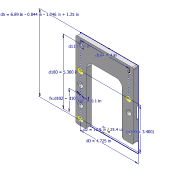
# Autodesk Inventor part: J002887
Saved by Autodesk Inventor 2012 SP2 (Build 160219200, 219)
## iProperties
Created: 2014-07-28
Material: ALUMINUM, 6061-T651
Vendor: HHMI: JFRC - ID&F
Document SubType Name: Modeling
Designer: arnoldj
Density: 2.7 g/cm^3
Part Number: J002887
Description: MPS Bottom Plate
Mass: 214.982 g
Surface Area: 270.982 cm^2
Volume: 79.623 cm^3
Project: P-194005
RuleStatus: InUse
AfterDocSave0: file://Part Number Cleaner
LAB/DEPT: SVOBODA (LAB)
REQUESTING SCIENTIST: PERON, SIMON
SURFACE ROUGHNESS: 63 Ra
DESIGN DEPARTMENT: HHMI: JFRC - ID&F
SPECIAL FINISH: ANODIZE PER MIL-A-8625F, TYPE II, CLASS 2 (BLACK)
ALTERED ITEM PART NUMBER: N/A
ALTERED ITEM VENDOR: N/A
ALTERED ITEM DESCRIPTION: N/A
Author: arnoldj
Revision Number: -
Autodesk Inventor part; units mm, degrees
ref_plane "Work Plane1 top of part" through (0, 0, 9.525) normal (0, 0, 1) x (1, 0, 0)
sketch "Sketch1" plane through (0, 0, 0) normal (0, 0, 1) x (1, 0, 0)
  line L0 (-60.0075, 146.25) -> (60.0075, 146.25)
  line L1 (60.0075, 146.25) -> (60.0075, -12.5)
  line L2 (-60.0075, -12.5) -> (-60.0075, 146.25)
  line L3 (-60.0075, -12.5) -> (60.0075, -12.5)
  point P0 (0, 0)
  point P1 (0, -3.5617)
  point P2 (0, 146.25)
  dimension "d0" = 120.015
  dimension "d2" = 12.5
  dimension "d5" = 158.75
  constraints: 8 end point, 2 perpendicular, 2 vertical alignment, 1 horizontal, 1 midpoint, 1 parallel
  measures "d0" distance of L1.end L2.start
  measures "d2" distance from line of L3 point (0, 0)
  measures "d5" distance of L2.start L0.start
extrude "Extrusion1" add sketch "Sketch1" along normal blind 9.525
sketch "Sketch2" plane through (0, 0, 0) normal (0, 0, 1) x (1, 0, 0)
  circle A0 centre (-50, 0) radius 3.175
  circle A1 centre (50, 86.36) radius 3.175
  circle A2 centre (-50, 86.36) radius 3.175
  point P0 (0, 0)
  point P1 (50, 35.56)
  dimension "d6" = 6.35
  dimension "d8" = 50
  dimension "d28" = 86.36
  dimension "d29" = 50
  dimension "d128" = 50.8
  constraints: 3 centre point, 1 equal radius, 1 horizontal alignment, 1 vertical alignment
  measures "d6" diameter of A0
  measures "d8" distance of point (0, 0) A0.centre
  measures "d28" distance of A0.centre A2.centre
  measures "d29" horizontal distance of point (0, 0) A1.centre
  measures "d128" distance of point (50, 35.56) A1.centre
hole "Hole1" at (-50, 0, 0) at (-50, 86.36, 0) at (50, 86.36, 0) direction (0, 0, 1) diameter 9.525 end through all
sketch "Sketch4" plane through (0, 0, 0) normal (0, 0, 1) x (1, 0, 0)
  line L0 (60.0075, -12.5) -> (-60.0075, -12.5) projected
  line L1 (0, 190.0524) -> (0, -46.2587) projected
  line L2 (-82.677, 0) -> (82.677, 0) projected
  line L3 (36.83, 110.944) -> (-36.83, 110.944)
  line L4 (-36.83, 110.944) -> (-36.83, -12.5)
  line L5 (36.83, 7.82) -> (60.0075, 7.82)
  line L6 (60.0075, 7.82) -> (60.0075, -12.5)
  line L7 (36.83, 7.82) -> (36.83, 110.944)
  line L8 (-36.83, -12.5) -> (60.0075, -12.5)
  line L9 (-60.0075, 146.25) -> (60.0075, 146.25) projected
  line L10 (0, -3.5649) -> (0, 156.2936)
  point P0 (0, 0)
  dimension "d30" = 123.444
  dimension "d31" = 20.32
  dimension "d32" = 35.306
  dimension "d112" = 73.66
  dimension "d132" = 36.83
  dimension "d133" = 36.83
  constraints: 14 end point, 3 point on line, 2 perpendicular, 1 collinear, 1 parallel, 1 symmetric about line
  measures "d30" distance of L3.end L4.end
  measures "d31" distance between parallel lines of L0 L5
  measures "d32" distance between parallel lines of L3 L9
  measures "d112" distance of L3.start L3.end
  measures "d132" distance between parallel lines of L1 L4
  measures "d133" distance between parallel lines of L7 L1
extrude "Extrusion3" cut sketch "Sketch4" along normal up to next
sketch "Sketch5" plane through (0, 0, 0) normal (0, 0, 1) x (1, 0, 0)
  circle A0 centre (-50, 86.36) radius 4.7625 projected
  circle A1 centre (50, 86.36) radius 4.7625 projected
  circle A2 centre (-50, 0) radius 4.7625 projected
  line L0 (-50, 86.36) -> (-50, 68.58) construction
  line L1 (-50, 0) -> (-50, 17.78) construction
  line L2 (50, 86.36) -> (50, 68.58) construction
  line L3 (-55.715, 74.295) -> (-44.285, 74.295)
  line L4 (-44.285, 74.295) -> (-44.285, 62.865)
  line L5 (-44.285, 62.865) -> (-55.715, 62.865)
  line L6 (-55.715, 62.865) -> (-55.715, 74.295)
  line L7 (-55.715, 23.495) -> (-44.285, 23.495)
  line L8 (-44.285, 23.495) -> (-44.285, 12.065)
  line L9 (-44.285, 12.065) -> (-55.715, 12.065)
  line L10 (-55.715, 12.065) -> (-55.715, 23.495)
  line L11 (44.285, 74.295) -> (55.715, 74.295)
  line L12 (55.715, 74.295) -> (55.715, 62.865)
  line L13 (55.715, 62.865) -> (44.285, 62.865)
  line L14 (44.285, 62.865) -> (44.285, 74.295)
  point P0 (0, 0)
  point P1 (-55.715, 68.58)
  point P2 (-50, 74.295)
  point P3 (-44.285, 17.78)
  point P4 (-50, 23.495)
  point P5 (55.715, 68.58)
  point P6 (50, 74.295)
  dimension "d36" = 17.78
  dimension "d38" = 11.43
  dimension "d39" = 11.43
  dimension "d63" = 50.8
  dimension "d97" = 17.78
  dimension "d98" = 17.78
  constraints: 30 end point, 12 equal length, 6 midpoint, 3 horizontal, 3 horizontal alignment, 3 perpendicular, 3 vertical alignment, 1 vertical
  measures "d36" distance of L1.start L1.end
  measures "d38" distance of L4.end L5.end
  measures "d39" distance of L5.end L3.start
  measures "d63" distance of L1.end L0.end
  measures "d97" distance of L0.start L0.end
  measures "d98" distance of L2.start L2.end
extrude "Extrusion4" [suppressed]
fillet "Fillet2" [suppressed]
fillet "Fillet3" radius 12.7 2 edges at (36.83, 110.944, 4.7625) (-36.83, 110.944, 4.7625)
fillet "Fillet4" radius 3.175 6 edges at (36.83, 7.82, 4.7625) (60.0075, 146.25, 4.7625) (-60.0075, 146.25, 4.7625) (-60.0075, -12.5, 4.7625) (-36.83, -12.5, 4.7625) (60.0075, 7.82, 4.7625)
sketch "Sketch9" plane through (0, 0, 9.525) normal (0, 0, 1) x (1, 0, 0)
  circle A0 centre (-50, 86.36) radius 4.7625 projected
  circle A1 centre (-50, 0) radius 4.7625 projected
  circle A2 centre (50, 86.36) radius 4.7625 projected
  line L0 (-50, 0) -> (-50, 140.9854) construction
  line L1 (50, 86.36) -> (50, 127.3454) construction
  circle A3 centre (-50, 43.18) radius 1.27 construction
  circle A4 centre (-50, 134.62) radius 1.27 construction
  circle A5 centre (51.6, 134.62) radius 1.5313 construction
  line L2 (-76.6675, 0) -> (76.6675, 0) construction
  point P0 (0, 0)
  dimension "d100" = 86.36
  dimension "d101" = 2.54
  dimension "d102" = 43.18
  dimension "d104" = 101.6
  dimension "d113" = 0
  dimension "d180" = 134.62
  constraints: 4 end point, 3 centre point, 2 point on line, 1 horizontal alignment, 1 parallel, 1 vertical
  measures "d100" distance of L0.start A0.centre
  measures "d101" diameter of A3
  measures "d102" distance from line of L2 A3.centre
  measures "d104" distance of A5.centre A4.centre
  measures "d113" distance of A4.centre point (-50, 134.62)
  measures "d180" distance from line of L2 point (-50, 134.62)
chamfer "Chamfer3" [suppressed]
chamfer "Chamfer4" distance 0.381 angle 45 6 edges at (-50, -4.7625, 9.525) (-50, 81.5975, 9.525) (50, 81.5975, 9.525) (-50, -4.7625, 0) (-50, 81.5975, 0) (50, 81.5975, 0)
sketch "Sketch10" plane through (0, 0, 0) normal (0, 0, 1) x (1, 0, 0)
  circle A0 centre (50, 86.36) radius 5.1435 construction
  line L0 (51.6, 134.62) -> (51.6, 24.6) construction
  line L1 (-76.6675, 0) -> (76.6675, 0) construction
  point P0 (0, 0)
  point P1 (-50, 134.62)
  point P2 (-50, 43.18)
  point P3 (-50, 43.18)
  point P4 (-50, 134.62)
  point P5 (-50, 134.62)
  dimension "d127" = 101.6
  dimension "d130" = 24.6
  dimension "d131" = 110.02
  constraints: 4 coincident, 2 end point, 1 vertical
  measures "d127" distance of L0.start point (-50, 134.62)
  measures "d130" distance from line of point (51.6, 24.6) L1
  measures "d131" distance of point (51.6, 24.6) L0.start
hole "Hole8 stdf holes flipped" at (51.6, 134.62, 0) at (-50, 134.62, 0) at (-50, 43.18, 0) at (51.6, 24.6, 0) direction (0, 0, 1) diameter 7.0358 end through all counterbore diameter 10.795 counterbore depth 6.35
sketch "Sketch11" plane through (0, 0, 0) normal (0, 0, 1) x (1, 0, 0)
  circle A0 centre (-50, 0) radius 4.7625 projected
  circle A1 centre (-50, 86.36) radius 4.7625 projected
  circle A2 centre (50, 86.36) radius 4.7625 projected
  point P0 (0, 0)
  point P1 (-50, 25.019)
  point P2 (-50, 61.341)
  point P3 (50, 61.341)
  dimension "d134" = 25.019
  dimension "d135" = 25.019
  dimension "d136" = 25.019
  measures "d134" distance of point (-50, 25.019) A0.centre
  measures "d135" distance of point (-50, 61.341) A1.centre
  measures "d136" distance of A2.centre point (50, 61.341)
hole "Hole9" at (50, 61.341, 0) at (-50, 61.341, 0) at (-50, 25.019, 0) direction (0, 0, 1) diameter 11.1125 end through all
sketch "Sketch13" plane through (0, 0, 0) normal (0, 0, -1) x (-1, 0, 0)
  circle A0 centre (50, 25.019) radius 5.5562 projected
  line L0 (60.0075, -9.325) -> (60.0075, 143.075) projected
  line L1 (39.205, 35.814) -> (60.0075, 35.814)
  line L2 (60.0075, 35.814) -> (60.0075, 14.224)
  line L3 (60.0075, 14.224) -> (39.205, 14.224)
  line L4 (39.205, 14.224) -> (39.205, 35.814)
  circle A1 centre (50, 61.341) radius 5.5562 projected
  line L5 (39.205, 72.136) -> (60.0075, 72.136)
  line L6 (60.0075, 72.136) -> (60.0075, 50.546)
  line L7 (60.0075, 50.546) -> (39.205, 50.546)
  line L8 (39.205, 50.546) -> (39.205, 72.136)
  point P0 (0, 0)
  dimension "d156" = 10.795
  dimension "d157" = 21.59
  dimension "d158" = 10.795
  dimension "d159" = 0
  dimension "d162" = 10.795
  dimension "d163" = 0
  dimension "d164" = 10.795
  dimension "d165" = 21.59
  constraints: 16 end point, 4 parallel, 2 horizontal, 2 perpendicular
  measures "d156" distance from line of L1 A0.centre
  measures "d157" distance of L3.end L1.start
  measures "d158" distance from line of L4 A0.centre
  measures "d159" distance between parallel lines of L0 L2
  measures "d162" distance from line of L8 A1.centre
  measures "d163" distance between parallel lines of L0 L6
  measures "d164" distance from line of A1.centre L5
  measures "d165" distance of L7.end L5.start
extrude "Extrusion5" cut sketch "Sketch13" against normal blind 2.54
sketch "Sketch14" plane through (0, 0, 2.54) normal (0, 0, -1) x (-1, 0, 0)
  circle A0 centre (50, 25.019) radius 5.5562 projected
  circle A1 centre (50, 25.019) radius 9.5 construction
  circle A2 centre (50, 61.341) radius 5.5562 construction
  circle A3 centre (50, 61.341) radius 9.5 construction
  point P0 (0, 0)
  point P1 (43.283, 68.059)
  point P2 (56.717, 68.059)
  point P3 (56.717, 54.623)
  point P4 (43.283, 54.623)
  point P5 (43.283, 31.737)
  point P6 (56.717, 31.737)
  point P7 (56.717, 18.301)
  point P8 (43.283, 18.301)
  dimension "d166" = 19
  dimension "d167" = 19
  dimension "d168" = 13.4341
  dimension "d169" = 13.436
  dimension "d170" = 13.4341
  dimension "d171" = 13.436
  constraints: 8 point on circle, 4 horizontal alignment, 4 vertical alignment, 2 centre point, 2 coincident
  measures "d166" diameter of A1
  measures "d167" diameter of A3
  measures "d168" distance of A3.start A3.end
  measures "d169" distance of point (43.283, 54.623) A3.start
  measures "d170" distance of A1.end A1.start
  measures "d171" distance of point (43.283, 18.301) A1.start
hole "Hole11" at (-43.283, 18.301, 2.54) at (-43.283, 31.737, 2.54) at (-56.717, 31.737, 2.54) at (-56.717, 18.301, 2.54) at (-43.283, 54.623, 2.54) at (-43.283, 68.059, 2.54) at (-56.717, 68.059, 2.54) at (-56.717, 54.623, 2.54) direction (0, 0, 1) diameter 2.0066 depth 6.35 tip angle 118
fillet "Fillet5" radius 1.5875 8 edges at (-39.205, 14.224, 1.27) (-39.205, 35.814, 1.27) (-39.205, 50.546, 1.27) (-39.205, 72.136, 1.27) (-60.0075, 50.546, 1.27) (-60.0075, 72.136, 1.27) (-60.0075, 35.814, 1.27) (-60.0075, 14.224, 1.27)
sketch "Sketch15" plane through (0, 0, 0) normal (0, 0, -1) x (-1, 0, 0)
  line L0 (-60.0075, 143.075) -> (-60.0075, 10.995) projected
  circle A0 centre (-50, 61.341) radius 5.5562 projected
  line L1 (-60.0075, 72.136) -> (-39.205, 72.136)
  line L2 (-39.205, 72.136) -> (-39.205, 50.546)
  line L3 (-39.205, 50.546) -> (-60.0075, 50.546)
  line L4 (-60.0075, 50.546) -> (-60.0075, 72.136)
  point P0 (0, 0)
  dimension "d181" = 21.59
  dimension "d182" = 10.795
  dimension "d183" = 10.795
  constraints: 8 end point, 2 parallel, 1 horizontal, 1 perpendicular, 1 point on line
  measures "d181" distance of L1.end L2.end
  measures "d182" distance from line of L1 A0.centre
  measures "d183" distance from line of A0.centre L2
extrude "Extrusion6" cut sketch "Sketch15" against normal blind 2.54
sketch "Sketch16" plane through (0, 0, 2.54) normal (0, 0, -1) x (-1, 0, 0)
  circle A0 centre (-50, 61.341) radius 5.5562 projected
  line L0 (-56.7176, 68.0584) -> (-43.2831, 68.0584) construction
  line L1 (-43.2831, 68.0584) -> (-43.2831, 54.6239) construction
  line L2 (-43.2831, 54.6239) -> (-56.7176, 54.6239) construction
  line L3 (-56.7176, 54.6239) -> (-56.7176, 68.0584) construction
  circle A1 centre (-50, 61.341) radius 9.5 construction
  point P0 (0, 0)
  dimension "d198" = 19
  dimension "d199" = 13.4345
  constraints: 8 end point, 5 coincident, 2 parallel, 2 perpendicular, 1 horizontal, 3 other
  measures "d199" distance of L0.start L0.end
hole "Hole12" at (43.2831, 68.0584, 2.54) at (43.2831, 54.6239, 2.54) at (56.7176, 54.6239, 2.54) at (56.7176, 68.0584, 2.54) direction (0, 0, 1) diameter 2.0066 depth 6.35 tip angle 118
fillet "Fillet6" radius 1.5875 4 edges at (60.0075, 72.136, 1.27) (39.205, 50.546, 1.27) (60.0075, 50.546, 1.27) (39.205, 72.136, 1.27)
equation "\"d29\" = d8"
body "Solid1"
